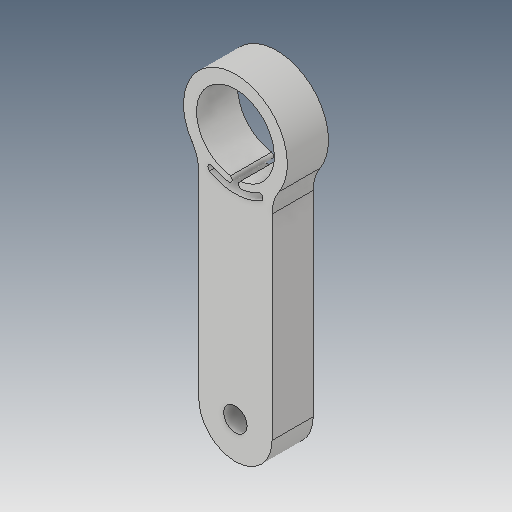
# Autodesk Inventor part: gripperPart4
Saved by Autodesk Inventor 2018 (Build 220112000, 112)
## iProperties
Created: 2020-01-19
Part Number: gripperPart4
Material: Generic
Document SubType Name: Modeling
Designer: anirudh
Density: 1 g/cm^3
Appearance: Default
Author: anirudh
Autodesk Inventor part; units mm, degrees
ref_plane "YZ Plane" through (0, 0, 0) normal (1, 0, 0) x (0, 1, 0)
ref_plane "XZ Plane" through (0, 0, 0) normal (0, 1, 0) x (-1, 0, 0)
ref_plane "XY Plane" through (0, 0, 0) normal (0, 0, 1) x (1, 0, 0)
sketch "Sketch1" plane through (0, 0, 0) normal (0, 0, 1) x (1, 0, 0)
  arc A0 (14.0648, 1.7612) -> (12.5672, 1.7612) centre (13.316, 7.7143) ccw
  arc A1 (14.0648, 1.7612) -> (12.5672, 1.7612) centre (13.316, 7.7143) ccw
  arc A2 (12.316, 0.7861) -> (12.5672, 1.7612) centre (12.2948, 1.3115) ccw
  arc A3 (12.3435, 0.788) -> (12.5672, 1.7612) centre (12.2948, 1.3115) ccw
  arc A4 (14.0648, 1.7612) -> (14.316, 0.7861) centre (14.3372, 1.3115) ccw
  arc A5 (9.753, 1.6889) -> (9.316, 0.7861) centre (9.5674, 1.2216) ccw
  arc A6 (9.8188, 1.6571) -> (9.316, 0.7861) centre (9.5674, 1.2216) ccw
  arc A7 (17.316, 0.7861) -> (16.816, 1.6522) centre (17.066, 1.2191) ccw
  arc A8 (17.316, 0.7861) -> (16.816, 1.6522) centre (17.066, 1.2191) ccw
  arc A9 (14.316, 0.7861) -> (16.816, 1.6522) centre (13.316, 7.7143) ccw
  arc A10 (9.316, 0.7861) -> (17.316, 0.7861) centre (13.316, 7.7143) ccw
  arc A11 (9.316, 0.7861) -> (17.316, 0.7861) centre (13.316, 7.7143) ccw
  arc A12 (9.8188, 1.6571) -> (12.3435, 0.788) centre (13.316, 7.7143) ccw
  arc A13 (14.0648, 1.7612) -> (14.316, 0.7861) centre (14.3372, 1.3115) ccw
  arc A14 (14.316, 0.7861) -> (16.816, 1.6522) centre (13.316, 7.7143) ccw
  line L0 (7.6645, -17.6857) -> (7.6645, 2.0521)
  line L1 (18.9675, -17.6857) -> (18.9675, 2.0521)
  arc A15 (9.316, 0.7861) -> (17.316, 0.7861) centre (13.316, 7.7143) ccw
  arc A16 (18.9675, 2.0521) -> (7.6645, 2.0521) centre (13.316, 7.7143) ccw
  line L2 (7.6645, -17.6857) -> (7.6645, -30.3857)
  line L3 (18.9675, -17.6857) -> (18.9675, -30.3857)
  arc A17 (7.6645, -30.3857) -> (18.9675, -30.3857) centre (13.316, -30.3857) ccw
  circle A18 centre (13.316, -30.3857) radius 1.8
  point P0 (18.0441, 0.8122)
  dimension "d10" = 3.6
  constraints: 43 point on circle, 19 centre point, 9 coincident, 8 end point, 3 vertical, 1 parallel
  measures "d10" diameter of A18
extrude "Extrusion2" add sketch "Sketch1" along normal blind 6.35
fillet "Fillet1" radius 6.35 2 edges at (18.9675, 2.0521, 3.175) (7.6645, 2.0521, 3.175)
body "Solid2"
